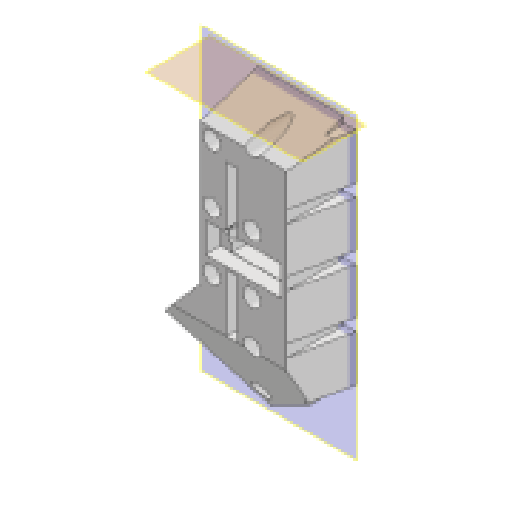
# Autodesk Inventor part: Wrist Base
Saved by Autodesk Inventor 2025.1 (Build 291241020, 241B)
## iProperties
Created: 2024-12-08
Part Number: Wrist Base
Material: Generic
Document SubType Name: Modeling
Designer: alexa
Density: 1 g/cm^3
Appearance: Default
Author: alexa
Autodesk Inventor part; units mm, degrees
ref_plane "YZ Plane" through (0, 0, 0) normal (1, 0, 0) x (0, 1, 0)
ref_plane "XZ Plane" through (0, 0, 0) normal (0, 1, 0) x (-1, 0, 0)
ref_plane "XY Plane" through (0, 0, 0) normal (0, 0, 1) x (1, 0, 0)
sketch "Sketch1" plane through (0, 0, 0) normal (0, 0, 1) x (1, 0, 0)
  line L0 (-19.3376, 7.8521) -> (11.9592, -19.9672) projected
  line L1 (38.1, -2.54) -> (11.9592, -19.9672) projected
  line L2 (-19.3376, 7.8521) -> (0, 29.6069) projected
  line L3 (0, 23.114) -> (0, 48.768) projected
  line L4 (0, 48.768) -> (0, 74.422) projected
  line L5 (0, 74.422) -> (0, 100.076) projected
  line L6 (0, 100.076) -> (38.1, 100.076) projected
  line L7 (38.1, 93.599) -> (38.1, 100.076) projected
  line L8 (38.1, 97.409) -> (43.18, 97.409) projected
  line L9 (43.18, 77.089) -> (43.18, 97.409) projected
  line L10 (38.1, 77.089) -> (43.18, 77.089) projected
  line L11 (38.1, 67.945) -> (38.1, 74.422) projected
  line L12 (38.1, 74.422) -> (38.1, 80.899) projected
  line L13 (38.1, 71.755) -> (43.18, 71.755) projected
  line L14 (43.18, 51.435) -> (43.18, 71.755) projected
  line L15 (38.1, 51.435) -> (43.18, 51.435) projected
  line L16 (38.1, 48.768) -> (38.1, 55.245) projected
  line L17 (38.1, 42.291) -> (38.1, 48.768) projected
  line L18 (38.1, 46.101) -> (43.18, 46.101) projected
  line L19 (43.18, 25.781) -> (43.18, 46.101) projected
  line L20 (38.1, 25.781) -> (43.18, 25.781) projected
  line L21 (38.1, 23.114) -> (38.1, 29.591) projected
  line L22 (38.1, 16.637) -> (38.1, 23.114) projected
  line L23 (38.1, 20.447) -> (43.18, 20.447) projected
  line L24 (43.18, 0.127) -> (43.18, 20.447) projected
  line L25 (38.1, 0.127) -> (43.18, 0.127) projected
  line L26 (38.1, -2.54) -> (38.1, 3.937) projected
  line L27 (-19.3376, 7.8521) -> (11.9592, -19.9672)
  line L28 (11.9592, -19.9672) -> (38.1, -2.54)
  line L29 (38.1, -2.54) -> (38.1, 0.127)
  line L30 (43.18, 0.127) -> (38.1, 0.127)
  line L31 (43.18, 0.127) -> (43.18, 20.447)
  line L32 (43.18, 20.447) -> (38.1, 20.447)
  line L33 (38.1, 20.447) -> (38.1, 25.781)
  line L34 (38.1, 25.781) -> (43.18, 25.781)
  line L35 (43.18, 25.781) -> (43.18, 46.101)
  line L36 (43.18, 46.101) -> (38.1, 46.101)
  line L37 (38.1, 46.101) -> (38.1, 51.435)
  line L38 (38.1, 51.435) -> (43.18, 51.435)
  line L39 (43.18, 51.435) -> (43.18, 71.755)
  line L40 (43.18, 71.755) -> (38.1, 71.755)
  line L41 (38.1, 71.755) -> (38.1, 77.089)
  line L42 (38.1, 77.089) -> (43.18, 77.089)
  line L43 (43.18, 77.089) -> (43.18, 97.409)
  line L44 (43.18, 97.409) -> (38.1, 97.409)
  line L45 (38.1, 97.409) -> (38.1, 100.076)
  line L46 (38.1, 100.076) -> (0, 100.076)
  line L47 (0, 100.076) -> (0, 29.6069)
  line L48 (0, 29.6069) -> (-19.3376, 7.8521)
  point P0 (0, 0)
  constraints: 44 end point, 17 collinear, 5 perpendicular
extrude "Extrusion1" add sketch "Sketch1" along normal blind 6.35
sketch "Sketch2" plane through (0, 0, 6.35) normal (0, 0, 1) x (1, 0, 0)
  line L0 (16.51, 66.675) -> (16.51, 56.515) projected
  line L1 (11.43, 66.675) -> (16.51, 66.675) projected
  line L2 (11.43, 56.515) -> (11.43, 66.675) projected
  line L3 (16.51, 56.515) -> (11.43, 56.515) projected
  line L4 (16.51, 82.169) -> (11.43, 82.169) projected
  line L5 (16.51, 92.329) -> (16.51, 82.169) projected
  line L6 (11.43, 92.329) -> (16.51, 92.329) projected
  line L7 (11.43, 82.169) -> (11.43, 92.329) projected
  line L8 (11.43, 30.861) -> (11.43, 41.021) projected
  line L9 (11.43, 41.021) -> (16.51, 41.021) projected
  line L10 (16.51, 41.021) -> (16.51, 30.861) projected
  line L11 (16.51, 30.861) -> (11.43, 30.861) projected
  line L12 (11.43, 15.367) -> (16.51, 15.367) projected
  line L13 (16.51, 15.367) -> (16.51, 5.207) projected
  line L14 (16.51, 5.207) -> (11.43, 5.207) projected
  line L15 (11.43, 5.207) -> (11.43, 15.367) projected
  point P0 (0, 0)
extrude "Extrusion2" cut sketch "Sketch2" against normal blind 6.35
sketch "Sketch3" plane through (0, 0, 6.35) normal (0, 0, 1) x (1, 0, 0)
  line L0 (16.51, 5.207) -> (11.43, 5.207) projected
  line L1 (11.43, 5.207) -> (11.43, 15.367) projected
  line L2 (11.43, 15.367) -> (16.51, 15.367) projected
  line L3 (16.51, 15.367) -> (16.51, 5.207) projected
  line L4 (38.1, 3.937) -> (33.02, 3.937) projected
  line L5 (33.02, 3.937) -> (33.02, 16.637) projected
  line L6 (33.02, 16.637) -> (38.1, 16.637) projected
  line L7 (38.1, 16.637) -> (38.1, 23.114) projected
  line L8 (0, 23.114) -> (38.1, 23.114) projected
  line L9 (0, -2.54) -> (0, 23.114) projected
  line L10 (0, -2.54) -> (38.1, -2.54) projected
  line L11 (38.1, -2.54) -> (38.1, 3.937) projected
  line L12 (16.51, 30.861) -> (11.43, 30.861) projected
  line L13 (11.43, 30.861) -> (11.43, 41.021) projected
  line L14 (11.43, 41.021) -> (16.51, 41.021) projected
  line L15 (16.51, 41.021) -> (16.51, 30.861) projected
  line L16 (38.1, 29.591) -> (33.02, 29.591) projected
  line L17 (33.02, 29.591) -> (33.02, 42.291) projected
  line L18 (33.02, 42.291) -> (38.1, 42.291) projected
  line L19 (38.1, 42.291) -> (38.1, 48.768) projected
  line L20 (0, 48.768) -> (38.1, 48.768) projected
  line L21 (0, 23.114) -> (0, 48.768) projected
  line L22 (0, 23.114) -> (38.1, 23.114) projected
  line L23 (38.1, 23.114) -> (38.1, 29.591) projected
  line L24 (16.51, 56.515) -> (11.43, 56.515) projected
  line L25 (11.43, 56.515) -> (11.43, 66.675) projected
  line L26 (11.43, 66.675) -> (16.51, 66.675) projected
  line L27 (16.51, 66.675) -> (16.51, 56.515) projected
  line L28 (38.1, 55.245) -> (33.02, 55.245) projected
  line L29 (33.02, 55.245) -> (33.02, 67.945) projected
  line L30 (33.02, 67.945) -> (38.1, 67.945) projected
  line L31 (38.1, 67.945) -> (38.1, 74.422) projected
  line L32 (0, 74.422) -> (38.1, 74.422) projected
  line L33 (0, 48.768) -> (0, 74.422) projected
  line L34 (0, 48.768) -> (38.1, 48.768) projected
  line L35 (38.1, 48.768) -> (38.1, 55.245) projected
  line L36 (16.51, 82.169) -> (11.43, 82.169) projected
  line L37 (11.43, 82.169) -> (11.43, 92.329) projected
  line L38 (11.43, 92.329) -> (16.51, 92.329) projected
  line L39 (16.51, 92.329) -> (16.51, 82.169) projected
  line L40 (38.1, 80.899) -> (33.02, 80.899) projected
  line L41 (33.02, 80.899) -> (33.02, 93.599) projected
  line L42 (33.02, 93.599) -> (38.1, 93.599) projected
  line L43 (38.1, 93.599) -> (38.1, 100.076) projected
  line L44 (0, 100.076) -> (38.1, 100.076) projected
  line L45 (0, 74.422) -> (0, 100.076) projected
  line L46 (0, 74.422) -> (38.1, 74.422) projected
  line L47 (38.1, 74.422) -> (38.1, 80.899) projected
  circle A0 centre (22.86, 35.941) radius 1.778
  circle A1 centre (22.86, 61.595) radius 1.778
  circle A2 centre (5.08, 87.249) radius 1.778
  circle A3 centre (5.08, 61.595) radius 1.778
  circle A4 centre (5.08, 35.941) radius 1.778
  circle A5 centre (5.08, 11.108) radius 1.778
  circle A6 centre (5.08, 87.249) radius 1.778 projected
  circle A7 centre (5.08, 61.595) radius 1.778 projected
  circle A8 centre (22.86, 61.595) radius 1.778 projected
  circle A9 centre (5.08, 35.941) radius 1.778 projected
  circle A10 centre (22.86, 35.941) radius 1.778 projected
  circle A11 centre (22.86, 16.764) radius 1.778
  circle A12 centre (22.86, 16.764) radius 1.778 projected
  circle A13 centre (22.86, 93.726) radius 1.778
  circle A14 centre (11.9592, -12.3472) radius 1.778
  point P0 (0, 0)
  point P1 (13.97, 15.367)
  point P2 (11.9592, -19.9672)
  dimension "d5" = 3.556
  dimension "d7" = 3.556
  dimension "d8" = 3.556
  dimension "d9" = 3.556
  dimension "d10" = 3.556
  dimension "d12" = 3.556
  dimension "d13" = 8.89
  dimension "d27" = 3.556
  dimension "d28" = 17.78
  dimension "d29" = 6.35
  dimension "d31" = 3.556
  dimension "d32" = 6.35
  dimension "d34" = 3.556
  dimension "d35" = 7.62
  constraints: 9 centre point, 6 vertical alignment, 2 horizontal alignment, 1 midpoint
  measures "d5" diameter of A5
  measures "d7" diameter of A0
  measures "d8" diameter of A4
  measures "d9" diameter of A3
  measures "d10" diameter of A1
  measures "d12" diameter of A2
  measures "d13" horizontal distance of point (13.97, 15.367) A5.centre
  measures "d27" diameter of A11
  measures "d28" horizontal distance of A5.centre A11.centre
  measures "d29" distance from line of L8 A11.centre
  measures "d31" diameter of A13
  measures "d32" distance from line of L44 A13.centre
  measures "d34" diameter of A14
  measures "d35" distance of point (11.959, -19.967) A14.centre
extrude "Extrusion3" cut sketch "Sketch3" against normal blind 6.35 contours A0 | A1 | A2 | A3 | A4 | A11 | A13 | A14
ref_plane "Work Plane1" through (0, 0, 2.54) normal (0, 0, -1) x (-1, 0, 0)
sketch "Sketch5" plane through (0, 0, 2.54) normal (0, 0, -1) x (-1, 0, 0)
  circle A0 centre (-22.86, 35.941) radius 1.778 projected
  circle A1 centre (-22.86, 35.941) radius 3.81
  circle A2 centre (-22.86, 61.595) radius 1.778 projected
  circle A3 centre (-22.86, 61.595) radius 3.81
  circle A4 centre (-5.08, 61.595) radius 1.778 projected
  circle A5 centre (-5.08, 61.595) radius 3.81
  circle A6 centre (-5.08, 35.941) radius 3.81
  circle A7 centre (-5.08, 87.249) radius 1.778 projected
  circle A8 centre (-5.08, 87.249) radius 3.81
  circle A9 centre (-22.86, 16.764) radius 1.778 projected
  circle A10 centre (-22.86, 16.764) radius 3.81
  circle A11 centre (-22.86, 93.726) radius 1.778 projected
  circle A12 centre (-22.86, 93.726) radius 3.81
  circle A13 centre (-11.9592, -12.3472) radius 1.778 projected
  circle A14 centre (-11.9592, -12.3472) radius 3.81
  point P0 (0, 0)
  point P1 (-5.08, 11.108)
  dimension "d17" = 7.62
  dimension "d19" = 7.62
  dimension "d20" = 7.62
  dimension "d22" = 7.62
  dimension "d30" = 7.62
  dimension "d33" = 7.62
  dimension "d36" = 7.62
  constraints: 8 centre point, 8 coincident
  measures "d17" diameter of A8
  measures "d19" diameter of A3
  measures "d20" diameter of A5
  measures "d22" diameter of A1
  measures "d30" diameter of A10
  measures "d33" diameter of A12
  measures "d36" diameter of A14
extrude "Extrusion4" cut sketch "Sketch5" against normal blind 6.35 contours A0 | A1 | A2 | A3 | A4 | A5 | A6 | A7 | A8 | A9 | A10 | A12 | A14
sketch "Sketch6" plane through (0, 0, 6.35) normal (0, 0, 1) x (1, 0, 0)
  line L0 (0, 29.6069) -> (-19.3376, 7.8521) projected
  line L1 (-19.3376, 7.8521) -> (11.9592, -19.9672) projected
  line L2 (11.9592, -19.9672) -> (38.1, -2.54) projected
  line L3 (38.1, -2.54) -> (38.1, 0.127) projected
  line L4 (38.1, 0.127) -> (43.18, 0.127) projected
  line L5 (43.18, 0.127) -> (43.18, 20.447) projected
  line L6 (43.18, 20.447) -> (38.1, 20.447) projected
  line L7 (38.1, 20.447) -> (38.1, 25.781) projected
  line L8 (38.1, 25.781) -> (43.18, 25.781) projected
  circle A0 centre (11.9592, -12.3472) radius 3.81 projected
  circle A1 centre (22.86, 16.764) radius 3.81 projected
  line L9 (43.18, 25.781) -> (43.18, 46.101) projected
  line L10 (43.18, 51.435) -> (43.18, 71.755) projected
  line L11 (38.1, 51.435) -> (43.18, 51.435) projected
  line L12 (38.1, 46.101) -> (38.1, 51.435) projected
  line L13 (43.18, 46.101) -> (38.1, 46.101) projected
  line L14 (43.18, 71.755) -> (38.1, 71.755) projected
  line L15 (38.1, 71.755) -> (38.1, 77.089) projected
  line L16 (38.1, 77.089) -> (43.18, 77.089) projected
  line L17 (43.18, 77.089) -> (43.18, 97.409) projected
  line L18 (43.18, 97.409) -> (38.1, 97.409) projected
  circle A2 centre (22.86, 16.764) radius 3.81 projected
  circle A3 centre (22.86, 61.595) radius 3.81 projected
  circle A4 centre (5.08, 87.249) radius 3.81 projected
  circle A5 centre (22.86, 93.726) radius 3.81 projected
  circle A6 centre (5.08, 35.941) radius 3.81 projected
  circle A7 centre (22.86, 35.941) radius 3.81 projected
  circle A8 centre (5.08, 61.595) radius 3.81 projected
  circle A9 centre (11.9592, -12.3472) radius 3.81 projected
  line L19 (16.51, 56.515) -> (11.43, 56.515) projected
  line L20 (11.43, 56.515) -> (11.43, 66.675) projected
  line L21 (11.43, 66.675) -> (16.51, 66.675) projected
  line L22 (16.51, 66.675) -> (16.51, 56.515) projected
  line L23 (11.43, 41.021) -> (16.51, 41.021) projected
  line L24 (16.51, 41.021) -> (16.51, 30.861) projected
  line L25 (16.51, 30.861) -> (11.43, 30.861) projected
  line L26 (11.43, 30.861) -> (11.43, 41.021) projected
  line L27 (11.43, 82.169) -> (11.43, 92.329) projected
  line L28 (11.43, 92.329) -> (16.51, 92.329) projected
  line L29 (16.51, 92.329) -> (16.51, 82.169) projected
  line L30 (16.51, 82.169) -> (11.43, 82.169) projected
  line L31 (16.51, 15.367) -> (16.51, 5.207) projected
  line L32 (16.51, 5.207) -> (11.43, 5.207) projected
  line L33 (11.43, 5.207) -> (11.43, 15.367) projected
  line L34 (11.43, 15.367) -> (16.51, 15.367) projected
  line L35 (43.18, 0.127) -> (43.18, 20.447) projected
  line L36 (43.18, 20.447) -> (38.1, 20.447) projected
  line L37 (38.1, 20.447) -> (38.1, 25.781) projected
  line L38 (38.1, 25.781) -> (43.18, 25.781) projected
  line L39 (43.18, 25.781) -> (43.18, 46.101) projected
  line L40 (43.18, 46.101) -> (38.1, 46.101) projected
  line L41 (38.1, 46.101) -> (38.1, 51.435) projected
  line L42 (38.1, 51.435) -> (43.18, 51.435) projected
  line L43 (43.18, 51.435) -> (43.18, 71.755) projected
  line L44 (43.18, 71.755) -> (38.1, 71.755) projected
  line L45 (38.1, 71.755) -> (38.1, 77.089) projected
  line L46 (38.1, 77.089) -> (43.18, 77.089) projected
  line L47 (43.18, 77.089) -> (43.18, 97.409) projected
  line L48 (43.18, 97.409) -> (38.1, 97.409) projected
  line L49 (38.1, 97.409) -> (38.1, 100.076) projected
  line L50 (38.1, 100.076) -> (0, 100.076) projected
  line L51 (0, 100.076) -> (0, 29.6069) projected
  line L52 (0, 29.6069) -> (-19.3376, 7.8521) projected
  line L53 (-19.3376, 7.8521) -> (11.9592, -19.9672) projected
  line L54 (11.9592, -19.9672) -> (38.1, -2.54) projected
  line L55 (38.1, -2.54) -> (38.1, 0.127) projected
  line L56 (38.1, 0.127) -> (43.18, 0.127) projected
  point P0 (0, 0)
extrude "Extrusion5" add sketch "Sketch6" along normal blind 19.05 contours L51 L50 L49 L18 L17 L16 L15 L14 L10 L11 L12 L13 L9 L8 L7 L6 L5 L4 L3 L2 L1 L0 | L27 L28 L29 L30 | L31 L32 L33 L34
sketch "Sketch7" plane through (43.18, 0.127, 0) normal (1, 0, 0) x (0, 0, -1)
  line L0 (-25.4, 29.4799) -> (-25.4, 7.7251) projected
  line L1 (-25.4, 15.4658) -> (-6.35, -20.0942)
  line L2 (0, -20.0942) -> (-25.4, -20.0942) projected
  line L3 (-6.35, -20.0942) -> (-25.4, -20.0942)
  line L4 (-25.4, -20.0942) -> (-25.4, 15.4658)
  line L5 (0, -20.0942) -> (0, -2.667) projected
  line L6 (0, 99.949) -> (-25.4, 99.949) projected
  line L7 (0, 99.949) -> (-25.4, 91.694)
  line L8 (-25.4, 99.949) -> (-25.4, 29.4799) projected
  line L9 (-25.4, 99.949) -> (-25.4, 91.694)
  line L10 (0, 99.949) -> (0, 29.4799) projected
  line L11 (-25.4, 99.949) -> (0, 99.949)
  point P0 (0, -0.127)
  dimension "d42" = 6.35
  dimension "d43" = 35.56
  dimension "d44" = 8.255
  constraints: 12 end point, 3 collinear, 3 point on line, 1 horizontal
  measures "d42" distance from line of L1.end L5
  measures "d43" distance from line of L2 L1.start
  measures "d44" distance of L6.end L7.end
extrude "Extrusion6" cut sketch "Sketch7" against normal blind 107.95
ref_plane "Work Plane2" through (38.1, 100.076, 0) normal (0, 1, 0) x (1, 0, 0)
sketch "Sketch8" plane through (38.1, 100.076, 0) normal (0, 1, 0) x (1, 0, 0)
  line L0 (0, -25.4) -> (5.08, -25.4) projected
  line L1 (5.08, 0) -> (5.08, -25.4) projected
  line L2 (0, -25.4) -> (5.08, 0)
  line L3 (5.08, 0) -> (5.08, -25.4)
  line L4 (5.08, -25.4) -> (0, -25.4)
  point P0 (-38.1, 0)
  constraints: 6 end point, 1 collinear, 1 perpendicular
extrude "Extrusion7" cut sketch "Sketch8" against normal blind 160.3375
sketch "Sketch10" plane through (0, 29.6069, 0) normal (-1, 0, 0) x (0, 0, 1)
  circle A0 centre (12.7, 44.8151) radius 1.778 projected
  point P0 (0, -29.6069)
extrude "Extrusion9" cut sketch "Sketch10" against normal blind 15.24
sketch "Sketch11" plane through (0, 0, 25.4) normal (0, 0, 1) x (1, 0, 0)
  line L0 (7.62, 42.418) -> (30.48, 42.418)
  line L1 (30.48, 42.418) -> (30.48, 55.118)
  line L2 (30.48, 55.118) -> (7.62, 55.118)
  line L3 (7.62, 55.118) -> (7.62, 42.418)
  line L4 (38.1, 46.101) -> (38.1, 51.435) projected
  point P0 (0, 0)
  point P1 (38.1, 48.768)
  dimension "d72" = 16.51
  dimension "d54" = 12.7
  dimension "d55" = 22.86
  dimension "d56" = 7.62
  dimension "d57" = 6.35
  constraints: 8 end point, 2 parallel, 1 horizontal, 1 midpoint, 1 perpendicular
  measures "d54" distance of L2.end L0.start
  measures "d55" distance of L1.end L2.end
  measures "d56" distance between parallel lines of L1 L4
  measures "d57" distance from line of point (38.1, 48.768) L0
extrude "Extrusion10" cut sketch "Sketch11" against normal blind 22.1742
sketch "Sketch12" plane through (0, 0, 25.4) normal (0, 0, 1) x (1, 0, 0)
  line L0 (6.223, 46.228) -> (16.51, 46.228)
  line L1 (16.51, 46.228) -> (16.51, 54.4996)
  line L2 (7.62, 51.308) -> (6.223, 51.308)
  line L3 (6.223, 51.308) -> (6.223, 46.228)
  line L4 (7.62, 42.418) -> (7.62, 55.118) projected
  line L5 (16.51, 56.515) -> (11.43, 56.515) projected
  line L6 (7.62, 51.308) -> (11.43, 56.515)
  line L7 (16.51, 56.515) -> (16.51, 54.4996)
  point P0 (0, 0)
  point P1 (6.223, 48.768)
  point P2 (7.62, 48.768)
  dimension "d60" = 5.08
  dimension "d61" = 1.397
  constraints: 12 end point, 2 midpoint, 2 parallel, 1 horizontal, 1 horizontal alignment, 1 perpendicular, 1 point on line, 1 vertical
  measures "d60" distance of L2.end L0.start
  measures "d61" distance between parallel lines of L3 L4
extrude "Extrusion11" cut sketch "Sketch12" against normal blind 23.5712
sketch "Sketch13" plane through (0, 0, 25.4) normal (0, 0, 1) x (1, 0, 0)
  circle A0 centre (33.02, 48.7758) radius 0.889
  circle A1 centre (5.08, 48.7758) radius 0.889
  line L0 (30.48, 42.418) -> (7.62, 42.418) projected
  point P0 (0, 0)
  point P1 (19.05, 42.418)
  dimension "d64" = 27.94
  dimension "d65" = 1.778
  dimension "d66" = 1.778
  dimension "d67" = 13.97
  constraints: 2 centre point, 1 horizontal alignment, 1 midpoint
  measures "d64" distance of A0.centre A1.centre
  measures "d65" diameter of A1
  measures "d66" diameter of A0
  measures "d67" horizontal distance of point (19.05, 42.418) A0.centre
extrude "Extrusion12" cut sketch "Sketch13" against normal blind 16.637
sketch "Sketch14" plane through (0, 0, 25.4) normal (0, 0, 1) x (1, 0, 0)
  line L0 (35.56, 42.1953) -> (2.54, 42.1953)
  line L1 (2.54, 42.1953) -> (2.54, 55.4033)
  line L2 (2.54, 55.4033) -> (35.56, 55.4033)
  line L3 (35.56, 55.4033) -> (35.56, 42.1953)
  line L4 (30.48, 42.418) -> (7.62, 42.418) projected
  point P0 (0, 0)
  point P1 (19.05, 42.418)
  dimension "d70" = 13.208
  dimension "d71" = 33.02
  dimension "d72" = 16.51
  constraints: 8 end point, 2 parallel, 1 horizontal, 1 midpoint, 1 perpendicular
  measures "d70" distance between parallel lines of L2 L0
  measures "d71" distance between parallel lines of L3 L1
  measures "d72" distance from line of point (19.05, 42.418) L3
extrude "Extrusion13" cut sketch "Sketch14" against normal blind 6.477
sketch "Sketch15" plane through (0, 0, 0) normal (0, 0, -1) x (-1, 0, 0)
  line L0 (-16.51, 15.367) -> (-11.43, 15.367) projected
  line L1 (-11.43, 82.169) -> (-16.51, 82.169) projected
  line L2 (-11.43, 30.861) -> (-16.51, 30.861) projected
  line L3 (-16.51, 15.367) -> (-11.43, 15.367)
  line L4 (-11.43, 15.367) -> (-11.43, 30.861)
  line L5 (-11.43, 30.861) -> (-16.51, 30.861)
  line L6 (-16.51, 30.861) -> (-16.51, 15.367)
  line L7 (-16.51, 82.169) -> (-11.43, 82.169)
  line L8 (-11.43, 82.169) -> (-11.43, 66.675)
  line L9 (-11.43, 66.675) -> (-16.51, 66.675)
  line L10 (-16.51, 66.675) -> (-16.51, 82.169)
  line L11 (-11.43, 66.675) -> (-16.51, 66.675) projected
  point P0 (0, 0)
  constraints: 16 end point, 4 parallel, 2 horizontal, 2 perpendicular, 2 point on line
extrude "Extrusion14" cut sketch "Sketch15" against normal blind 66.675
chamfer "Chamfer1" distance 2.54 angle 45 4 edges at (11.43, 87.249, 6.35) (16.51, 87.249, 6.35) (16.51, 10.287, 6.35) (11.43, 10.287, 6.35)
equation "\"d7\" = d5"
equation "\"d8\" = d5"
equation "\"d9\" = d5"
equation "\"d10\" = d5"
equation "\"d12\" = d5"
equation "\"d13\" = 0.5 * d28"
equation "\"d34\" = d5"
equation "\"d19\" = d17"
equation "\"d20\" = d17"
equation "\"d22\" = d17"
equation "\"d33\" = d17"
equation "\"d36\" = d30"
equation "\"d72\" = 0.5 * d71"
equation "\"d57\" = 0.5 * d54"
equation "\"d67\" = 0.5 * d64"
body "Solid1"
